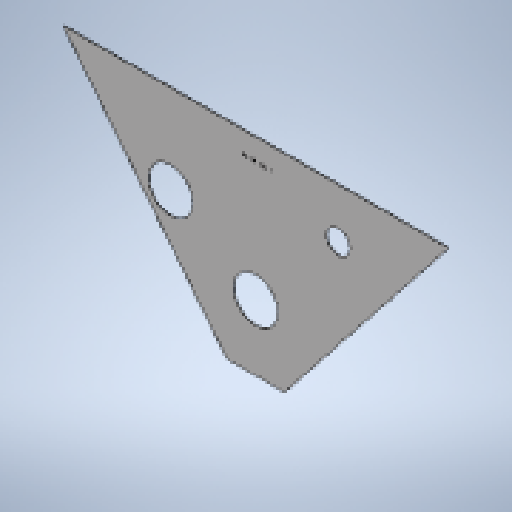
# Autodesk Inventor part: MSC 701 face 1
Saved by Autodesk Inventor 2025 (Build 290162010, 162A)
## iProperties
Created: 2024-06-08
Part Number: MSC 701 face 1
Material: Stainless Steel
Document SubType Name: Sheet Metal
Designer: admin
Density: 8 g/cm^3
Sheet Metal Rule: AISI304 2mm Die16
Appearance: Default
Stock Number: МОО 701 морда 1
Flat Pattern Width: 79 cm
Flat Pattern Length: 147.018 cm
Flat Pattern Area: 11614.4 cm^2
Sheet Metal Width: 790,000 mm
Sheet Metal Length: 1470,181 mm
Sheet Metal Area: 1161443,222 mm^2
Author: admin
Autodesk Inventor part; units mm, degrees
ref_plane "YZ Plane" through (0, 0, 0) normal (1, 0, 0) x (0, 1, 0)
ref_plane "XZ Plane" through (0, 0, 0) normal (0, 1, 0) x (-1, 0, 0)
ref_plane "XY Plane" through (0, 0, 0) normal (0, 0, 1) x (1, 0, 0)
sketch "Sketch1" plane through (0, 0, 0) normal (0, 1, 0) x (-1, 0, 0)
  line L0 (0, 790) -> (0, 0)
  line L1 (735.0906, 788) -> (735.0906, 790)
  line L2 (735.0906, 790) -> (0, 790)
  line L3 (735.0906, 788) -> (110, 0)
  line L4 (110, 0) -> (0, 0)
  point P0 (0, 678)
  dimension "d1" = 735.0906
  dimension "d2" = 2
  dimension "d5" = 128.424
  dimension "d6" = 110
  dimension "d9" = 790
  measures "d1" distance of L1.end L0.start
  measures "d2" distance of L1.start L1.end
  measures "d5" angle of L4 L3
  measures "d6" distance of L0.end L3.end
  measures "d9" distance of L0.start L0.end
extrude "Plate1" add sketch "Sketch1" along normal blind 2
mirror "Mirror1" about plane through (0, 0, 0) normal (1, 0, 0) of "Plate1"
sketch "Sketch2" plane through (0, 0, 0) normal (0, -1, 0) x (1, 0, 0)
  line L0 (-110, 0) -> (110, 0) construction
  line L1 (-110, 0) -> (-735.0906, 788) construction
  circle A0 centre (-325, 450) radius 84.5
  line L2 (110, 0) -> (735.0906, 788) construction
  circle A1 centre (0, 250) radius 84.5
  circle A2 centre (315, 600) radius 45
  line L3 (-110, 0) -> (110, 0) construction
  line L4 (-240.5, 450) -> (-240.5, 164.5105) construction
  line L5 (-84.5, 250) -> (-84.5, 0) construction
  line L6 (84.5, 250) -> (84.5, 0) construction
  line L7 (270, 600) -> (270, 0) construction
  line L8 (-325, 534.5) -> (270, 534.5) construction
  line L9 (-325, 365.5) -> (270, 365.5) construction
  line L10 (0, 334.5) -> (270, 334.5) construction
  line L11 (315, 555) -> (270, 555) construction
  line L12 (-735.0906, 790) -> (735.0906, 790) projected
  line L13 (-735.0906, 788) -> (-735.0906, 790) projected
  line L14 (735.0906, 788) -> (735.0906, 790) projected
  point P0 (0, 0)
  point P1 (0, 0)
  point P2 (0, 0)
  point P3 (0, 0)
  point P4 (-84.5, 144.3746)
  point P5 (0, 0)
  point P6 (0, 0)
  dimension "d13" = 169
  dimension "d16" = 250
  dimension "d17" = 450
  dimension "d18" = 325
  dimension "d19" = 31
  dimension "d20" = 90
  dimension "d21" = 156
  dimension "d23" = 315
  dimension "d24" = 600
  constraints: 16 end point, 8 point on circle, 8 tangent, 6 point on line, 4 perpendicular, 3 centre point, 2 horizontal, 2 vertical, 1 equal radius, 1 midpoint, 1 vertical alignment, 8 other
  measures "d13" diameter of A0
  measures "d16" distance from line of L0 A1.centre
  measures "d17" distance from line of L0 A0.centre
  measures "d18" horizontal distance of A0.centre point (0, 0)
  measures "d19" distance between parallel lines of L10 L9
  measures "d20" diameter of A2
  measures "d21" distance from line of point (-84.5, 144.375) L4
  measures "d23" horizontal distance of point (0, 0) A2.centre
  measures "d24" distance from line of L0 A2.centre
extrude "Extrusion1" cut sketch "Sketch2" against normal through all
sketch "Sketch3" plane through (0, 0, 0) normal (0, -1, 0) x (1, 0, 0)
  line L0 (-53.9958, 701.8167) -> (-53.9958, 713.8167) construction
  line L1 (-53.9958, 713.8167) -> (56.0042, 713.8167) construction
  line L2 (56.0042, 713.8167) -> (56.0042, 701.8167) construction
  line L3 (56.0042, 701.8167) -> (-53.9958, 701.8167) construction
  point P0 (0, 0)
  point P1 (1.0042, 701.8167)
  dimension "d25" = 12
  dimension "d26" = 110
  constraints: 1 midpoint, 2 other
  measures "d25" distance of L1.end L2.end
  measures "d26" distance between parallel lines of L0 L2
mark "Mark1"
equation "\"d3\" = Thickness"
equation "\"BendReliefWidth\" = Thickness"
equation "\"BendReliefDepth\" = 0.5 * Thickness"
equation "\"CornerReliefSize\" = 4 * Thickness"
equation "\"MinimumRemnant\" = 2 * Thickness"
equation "\"GapSize\" = Thickness"
equation "\"Thickness\" = 2"
body "Solid1"
